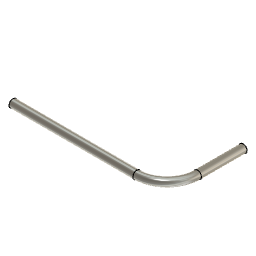
Free stream tube (Autodesk Fusion 360 design; units mm, degrees)
Autodesk Fusion 360 part; units mm, degrees
sketch "Sketch1" plane through (0, 0, 0) normal (1, 0, 0) x (0, 1, 0)
  circle A0 centre (0, 0) radius 1.3
  circle A1 centre (0, 0) radius 1.1476
  dimension "d1" = 2.6
  dimension "d2" = 2.2952
  constraint coincident A0.centre A1.centre
  measures "d1" diameter of A0
  measures "d2" diameter of A1
sketch "Sketch2" plane through (0, 0, 0) normal (0, 0, 1) x (1, 0, 0)
  line L0 (0, 0) -> (40.8, 0)
  line L1 (50.8, 10) -> (50.8, 25)
  arc A0 (40.8, 0) -> (50.8, 10) centre (40.8, 10) ccw
  point P0 (50.8, 0)
  dimension "d3" = 50.8
  dimension "d4" = 25
  dimension "d5" = 10
  constraint coincident L0.start origin
  constraint horizontal L0
  constraint perpendicular L0 L1
  constraint coincident P0 L0
  constraint coincident P0 L1
  constraint tangent L0 A0
  constraint tangent L1 A0
  measures "d3" distance of L0.start P0
  measures "d4" distance of P0 L1.end
  measures "d5" radius of A0
sweep "Sweep1" add profiles "Sketch1" path "Sketch2" along L0 A0 L1 section 1
equation "d2 = d1 - 0.012 in"
